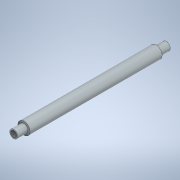
# Autodesk Inventor part: Guais de Soporte de Motor
Saved by Autodesk Inventor 2020 (Build 240168000, 168)
## iProperties
Created: 2020-05-16
Part Number: Guais de Soporte de Motor
Material: Steel, High Strength, Low Alloy
Document SubType Name: Modeling
Designer: Dante
Density: 7.85 g/cm^3
Appearance: Zinc
Mass: 122.074 g
Surface Area: 68.2354 cm^2
Volume: 15.5509 cm^3
Author: Dante
Autodesk Inventor part; units mm, degrees
ref_plane "YZ Plane" through (0, 0, 0) normal (1, 0, 0) x (0, 1, 0)
ref_plane "XZ Plane" through (0, 0, 0) normal (0, 1, 0) x (-1, 0, 0)
ref_plane "XY Plane" through (0, 0, 0) normal (0, 0, 1) x (1, 0, 0)
sketch "Sketch1" plane through (0, 0, 0) normal (0, 0, 1) x (1, 0, 0)
  circle A0 centre (0, 0) radius 6
  circle A1 centre (0, 0) radius 3
  dimension "d0" = 12
  dimension "d1" = 6
  constraints: 2 centre point, 2 coincident
  measures "d0" diameter of A0
  measures "d1" diameter of A1
extrude "Extrusion1" add sketch "Sketch1" along normal blind 150 contours A0 | A1
sketch "Sketch2" plane through (0, 0, 150) normal (0, 0, 1) x (1, 0, 0)
  circle A0 centre (0, 0) radius 3
  dimension "d4" = 6
  constraints: 1 centre point, 1 coincident
  measures "d4" diameter of A0
extrude "Extrusion2" cut sketch "Sketch2" against normal blind 25
extrude "Extrusion3" cut sketch "Sketch1" along normal blind 25 contours A1
thread "Thread1" size "M6x1" class "6H" standard "ANSI Metric M Profile" length 348
thread "Thread2" size "M6x1" class "6H" standard "ANSI Metric M Profile" length 348
sketch "Boceto3" plane through (0, 0, 150) normal (0, 0, 1) x (1, 0, 0)
  circle A0 centre (0, 0) radius 6
  circle A1 centre (0, 0) radius 4
  dimension "d13" = 8
  constraints: 2 centre point, 2 coincident
  measures "d13" diameter of A1
sketch "Boceto4" plane through (0, 0, 0) normal (0, 0, -1) x (-1, 0, 0)
  circle A0 centre (0, 0) radius 6
  circle A1 centre (0, 0) radius 4
  dimension "d14" = 8
  constraints: 2 centre point, 2 coincident
  measures "d14" diameter of A1
extrude "Extrusión4" cut sketch "Boceto4" against normal blind 10
extrude "Extrusión5" cut sketch "Boceto3" against normal blind 10
body "Solid1"
